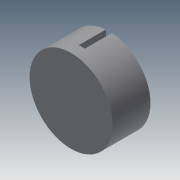
# Autodesk Inventor part: speaker_base
Saved by Autodesk Inventor 2015 (Build 190159000, 159)
## iProperties
Created: 2018-01-20
Part Number: speaker_base
Material: Generic
Document SubType Name: Modeling
Designer: rissa
Density: 1 g/cm^3
Appearance: Default
Author: rissa
Autodesk Inventor part; units mm, degrees
ref_plane "YZ Plane" through (0, 0, 0) normal (1, 0, 0) x (0, 1, 0)
ref_plane "XZ Plane" through (0, 0, 0) normal (0, 1, 0) x (-1, 0, 0)
ref_plane "XY Plane" through (0, 0, 0) normal (0, 0, 1) x (1, 0, 0)
sketch "Sketch1" plane through (0, 0, 0) normal (0, 0, 1) x (1, 0, 0)
  circle A0 centre (0, 0) radius 27.5
  dimension "d0" = 55
  constraints: 1 centre point, 1 coincident
  measures "d0" diameter of A0
extrude "Extrusion1" add sketch "Sketch1" along normal blind 25
sketch "Sketch2" plane through (0, 0, 0) normal (0, 0, -1) x (-1, 0, 0)
  line L0 (6.1, -11.3) -> (-6.1, -11.3)
  line L1 (-6.1, -11.3) -> (-6.1, 11.3)
  line L2 (-6.1, 11.3) -> (6.1, 11.3)
  line L3 (6.1, 11.3) -> (6.1, -11.3)
  circle A0 centre (0, 0) radius 27.5 projected
  dimension "d4" = 12.2
  dimension "d5" = 55
  dimension "d6" = 22.6
  dimension "d7" = 6.1
  dimension "d8" = 11.3
  constraints: 8 end point, 2 parallel, 1 horizontal, 1 perpendicular
  measures "d4" distance between parallel lines of L1 L3
  measures "d5" diameter of A0
  measures "d6" distance between parallel lines of L2 L0
  measures "d7" distance from line of L1 point (0, 0)
  measures "d8" distance from line of L0 point (0, 0)
extrude "Extrusion2" cut sketch "Sketch2" against normal blind 23 contours L0 L1 L2 L3
sketch "Sketch3" plane through (0, 0, 0) normal (0, 0, -1) x (-1, 0, 0)
  line L0 (-6.1, 11.3) -> (6.1, 11.3) projected
  line L1 (6.1, -11.3) -> (-6.1, -11.3) projected
  line L2 (6.1, 11.3) -> (6.1, -11.3) projected
  line L3 (-6.1, -11.3) -> (-6.1, 11.3) projected
  line L4 (6.1, -16.5) -> (-6.1, -16.5)
  line L5 (-6.1, -16.5) -> (-6.1, 16.5)
  line L6 (-6.1, 16.5) -> (6.1, 16.5)
  line L7 (6.1, 16.5) -> (6.1, -16.5)
  point P0 (0, 0)
  dimension "d11" = 22.6
  dimension "d12" = 12.2
  dimension "d13" = 5.2
  dimension "d14" = 5.2
  constraints: 8 end point, 2 parallel, 1 horizontal, 1 perpendicular
  measures "d11" distance between parallel lines of L0 L1
  measures "d12" distance between parallel lines of L2 L3
  measures "d13" distance between parallel lines of L1 L4
  measures "d14" distance between parallel lines of L0 L6
extrude "Extrusion3" cut sketch "Sketch3" against normal blind 6 contours L5 L6 L7 L0 | L1 L7 L4 L5
sketch "Sketch4" plane through (0, 0, 0) normal (0, 0, -1) x (-1, 0, 0)
  line L0 (-6.1, -16.5) -> (-6.1, 16.5) projected
  line L1 (6.1, 16.5) -> (6.1, -16.5) projected
  line L2 (-6.1, 16.5) -> (6.1, 16.5) projected
  line L3 (6.1, -16.5) -> (-6.1, -16.5) projected
  line L4 (6.1, 11.3) -> (-6.1, 11.3) projected
  line L5 (-6.1, -11.3) -> (6.1, -11.3) projected
  line L6 (-6.1, 16.5) -> (6.1, 16.5) projected
  line L7 (2, 16.5) -> (2, 27.4272)
  circle A0 centre (0, 0) radius 27.5 projected
  line L8 (-2, 16.5) -> (-2, 27.4272)
  arc A1 (2, 27.4272) -> (-2, 27.4272) centre (0, 0) ccw
  line L9 (2, 16.5) -> (2, 11.3)
  line L10 (-2, 16.5) -> (-2, 11.3)
  dimension "d17" = 12.2
  dimension "d18" = 33
  dimension "d19" = 22.6
  dimension "d20" = 4
  dimension "d21" = 4.1
  constraints: 8 end point, 4 perpendicular, 4 point on circle, 4 point on line, 1 centre point, 1 concentric
  measures "d17" distance between parallel lines of L0 L1
  measures "d18" distance between parallel lines of L2 L3
  measures "d19" distance between parallel lines of L4 L5
  measures "d20" distance between parallel lines of L8 L7
  measures "d21" distance from line of L0.end L8
extrude "Extrusion4" cut sketch "Sketch4" against normal blind 18 contours L10 L2 L9 L4 | L8 A0 L7 L2
hole "Hole2" at (21.1, -0.2, 0) direction (0, 0, 1) diameter 1.567 depth 4.2 tip angle 118 thread size "M2x0.4" class "6H" standard "ANSI Metric M Profile"
hole "Hole3" at (-21.1, -0.2, 0) direction (0, 0, 1) diameter 1.567 depth 4.2 tip angle 118 thread size "M2x0.4" class "6H" standard "ANSI Metric M Profile"
body "Solid1"
